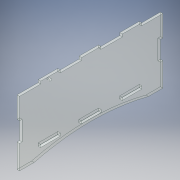
# Autodesk Inventor part: Enclosure Back
Saved by Autodesk Inventor 2018 (Build 220112000, 112)
## iProperties
Created: 2017-12-06
Part Number: Enclosure Back
Material: Glass
Document SubType Name: Modeling
Designer: Andrew
Density: 2.18 g/cm^3
Appearance: Clear
Author: Andrew
Autodesk Inventor part; units mm, degrees
ref_plane "YZ Plane" through (0, 0, 0) normal (1, 0, 0) x (0, 1, 0)
ref_plane "XZ Plane" through (0, 0, 0) normal (0, 1, 0) x (-1, 0, 0)
ref_plane "XY Plane" through (0, 0, 0) normal (0, 0, 1) x (1, 0, 0)
derived "Enclosure Top.ipt"
sketch "Sketch2" plane through (0, 0, 0) normal (0, 1, 0) x (-1, 0, 0)
  line L0 (-41.402, 93.7895) -> (-41.402, -93.7895)
  line L1 (-41.402, -93.7895) -> (41.402, -93.7895)
  line L2 (41.402, -93.7895) -> (41.402, 93.7895)
  line L3 (41.402, 93.7895) -> (-41.402, 93.7895)
  line L4 (33.576, -93.7895) -> (7.826, -93.7895)
  line L5 (7.826, -93.7895) -> (7.826, -90.4875)
  line L6 (7.826, -90.4875) -> (33.576, -90.4875)
  line L7 (33.576, -90.4875) -> (33.576, -93.7895)
  line L8 (-7.826, -93.7895) -> (-33.576, -93.7895)
  line L9 (-33.576, -93.7895) -> (-33.576, -90.4875)
  line L10 (-33.576, -90.4875) -> (-7.826, -90.4875)
  line L11 (-7.826, -90.4875) -> (-7.826, -93.7895)
  line L12 (0, -131.3053) -> (0, 131.3053)
  line L13 (-66.8528, 0) -> (66.8528, 0)
  line L14 (-41.402, -66.2073) -> (-38.1, -66.2073)
  line L15 (-38.1, -66.2073) -> (-38.1, -40.4572)
  line L16 (-38.1, -40.4572) -> (-41.402, -40.4572)
  line L17 (-41.402, -40.4572) -> (-41.402, -66.2073)
  line L18 (-41.402, -12.875) -> (-38.1, -12.875)
  line L19 (-38.1, -12.875) -> (-38.1, 12.875)
  line L20 (-38.1, 12.875) -> (-41.402, 12.875)
  line L21 (-41.402, 12.875) -> (-41.402, -12.875)
  line L22 (-41.402, 40.4572) -> (-38.1, 40.4572)
  line L23 (-38.1, 40.4572) -> (-38.1, 66.2073)
  line L24 (-38.1, 66.2073) -> (-41.402, 66.2073)
  line L25 (-41.402, 66.2073) -> (-41.402, 40.4572)
  line L26 (38.1, 50.3478) -> (36.5506, 50.3477)
  line L27 (36.5506, 50.3477) -> (36.5506, 56.3167)
  line L28 (36.5506, 56.3167) -> (38.1, 56.3167)
  line L29 (38.1, 56.3167) -> (38.1, 50.3478)
  point P0 (0, 0)
  point P1 (20.701, -90.4875)
  point P2 (-38.1, -53.3322)
  point P3 (36.5506, 53.3322)
  point P4 (-38.1, 53.3322)
sketch "Sketch3" plane through (0, 0, 0) normal (1, 0, 0) x (0, 1, 0)
  line L0 (0, 93.7895) -> (0, -93.7895) projected
  line L1 (0, 93.7895) -> (-87.817, 93.7895)
  line L2 (-87.817, -93.7895) -> (0, -93.7895)
  line L3 (-3.302, 93.7895) -> (-3.302, -93.7895) construction
  line L4 (-71.592, 93.7895) -> (-71.592, -93.7895) construction
  line L5 (-75.117, 93.7895) -> (-75.117, -93.7895) construction
  line L6 (-87.817, 93.7895) -> (-87.817, 74.7395)
  line L7 (-87.817, -93.7895) -> (-87.817, -74.7395)
  arc A0 (-87.817, -74.7395) -> (-87.817, 74.7395) centre (-376.2825, 0) ccw
  line L8 (-71.592, 66.2073) -> (-75.117, 66.2073)
  line L9 (-75.117, 66.2073) -> (-75.117, 40.4573)
  line L10 (-75.117, 40.4573) -> (-71.592, 40.4573)
  line L11 (-71.592, 40.4573) -> (-71.592, 66.2073)
  line L12 (-71.592, 12.875) -> (-75.117, 12.875)
  line L13 (-75.117, 12.875) -> (-75.117, -12.875)
  line L14 (-75.117, -12.875) -> (-71.592, -12.875)
  line L15 (-71.592, -12.875) -> (-71.592, 12.875)
  line L16 (-71.592, -40.4573) -> (-75.117, -40.4573)
  line L17 (-75.117, -40.4573) -> (-75.117, -66.2073)
  line L18 (-75.117, -66.2073) -> (-71.592, -66.2073)
  line L19 (-71.592, -66.2073) -> (-71.592, -40.4573)
  line L20 (-451.5389, 0) -> (75.2565, 0) projected
  circle A1 centre (-4.826, 53.3322) radius 1.4605
  point P0 (0, 0)
  point P1 (0, -53.3322)
  point P2 (-71.592, -53.3323)
  dimension "d10" = 3.302
  dimension "d12" = 71.592
  dimension "d13" = 3.525
  dimension "d15" = 19.05
  dimension "d16" = 12.7
  dimension "d17" = 25.75
  dimension "d20" = 3.175
  dimension "d22" = 40.4573
  dimension "d23" = 2.921
  dimension "d24" = 4.826
  constraints: 38 end point, 12 point on line, 6 parallel, 6 perpendicular, 4 collinear, 4 horizontal, 2 centre point, 2 point on circle, 2 vertical, 1 horizontal alignment, 1 midpoint, 2 other
  measures "d10" distance between parallel lines of L3 L0
  measures "d12" distance between parallel lines of L4 L0
  measures "d13" distance between parallel lines of L5 L4
  measures "d15" distance of L2.start L7.end
  measures "d16" distance between parallel lines of L7 L5
  measures "d17" distance of L10.end L8.start
  measures "d20" distance edge to line of A0 L5
  measures "d22" distance from line of L1 A1.centre
  measures "d23" diameter of A1
  measures "d24" distance from line of L0 A1.centre
extrude "Extrusion1" add sketch "Sketch3" along normal blind 3.302 contours L0 L20 L15 L12 L13 A0 L6 L1 | L0 L2 L7 A0 L20 L13 L14 L15
sketch "Sketch4" plane through (0, 0, 0) normal (1, 0, 0) x (0, 1, 0)
  line L0 (-451.5389, 0) -> (75.2565, 0) projected
  line L1 (0, 93.7895) -> (-87.817, 93.7895) projected
  line L2 (-87.817, -93.7895) -> (0, -93.7895) projected
  line L3 (0, 93.7895) -> (0, -93.7895) projected
  line L4 (0, -40.6323) -> (-3.302, -40.6323)
  line L5 (-3.302, -40.6323) -> (-3.302, -12.7)
  line L6 (-3.302, -12.7) -> (0, -12.7)
  line L7 (0, -12.7) -> (0, -40.6323)
  line L8 (0, -66.0323) -> (-3.302, -66.0323)
  line L9 (-3.302, -66.0323) -> (-3.302, -93.7895)
  line L10 (-3.302, -93.7895) -> (0, -93.7895)
  line L11 (0, -93.7895) -> (0, -66.0323)
  line L12 (0, 12.7) -> (-3.302, 12.7)
  line L13 (-3.302, 12.7) -> (-3.302, 40.6323)
  line L14 (-3.302, 40.6323) -> (0, 40.6323)
  line L15 (0, 40.6323) -> (0, 12.7)
  line L16 (0, 66.0323) -> (-3.302, 66.0323)
  line L17 (-3.302, 66.0323) -> (-3.302, 93.7895)
  line L18 (-3.302, 93.7895) -> (0, 93.7895)
  line L19 (0, 93.7895) -> (0, 66.0323)
  line L20 (-87.817, -93.7895) -> (-87.817, -74.7395) projected
  arc A0 (-87.817, -74.7395) -> (-87.817, 74.7395) centre (-376.2825, 0) ccw projected
  line L21 (-87.817, 93.7895) -> (-87.817, 74.7395) projected
  line L22 (-31.0335, 93.7895) -> (-56.7835, 93.7895)
  line L23 (-56.7835, 93.7895) -> (-56.7835, 90.4875)
  line L24 (-56.7835, 90.4875) -> (-31.0335, 90.4875)
  line L25 (-31.0335, 90.4875) -> (-31.0335, 93.7895)
  line L26 (-71.592, 93.7895) -> (-71.592, -93.7895) construction
  line L27 (-75.117, 93.7895) -> (-75.117, -93.7895) construction
  line L28 (-31.0335, -93.7895) -> (-56.7835, -93.7895)
  line L29 (-56.7835, -93.7895) -> (-56.7835, -90.4875)
  line L30 (-56.7835, -90.4875) -> (-31.0335, -90.4875)
  line L31 (-31.0335, -90.4875) -> (-31.0335, -93.7895)
  point P0 (0, 0)
  point P1 (0, -53.3322)
  point P2 (-43.9085, 90.4875)
  point P3 (-43.9085, 93.7895)
  dimension "d4" = 25.4
  dimension "d5" = 25.4
  dimension "d6" = 25.4
  dimension "d7" = 3.302
  dimension "d8" = 12.7
  dimension "d21" = 25.75
  constraints: 48 end point, 12 parallel, 10 point on line, 8 perpendicular, 6 horizontal, 3 collinear, 2 midpoint, 1 vertical alignment, 2 other
  measures "d4" distance between parallel lines of L16 L14
  measures "d5" distance between parallel lines of L6 L12
  measures "d6" distance between parallel lines of L8 L4
  measures "d7" distance of L16.start L16.end
  measures "d8" distance from line of point (0, -53.332) L4
  measures "d21" distance of L23.end L24.end
derived "Wood Rail.ipt"
extrude "Extrusion2" cut sketch "Sketch4" along normal blind 3.302 contours L12 L13 L14 L3 | L3 L4 L5 L6 | L29 L30 L31 L2 | L1 L25 L24 L23 | L16 L17 L1 L3 | L3 L2 L9 L8
equation "\"d10\" = encThick"
equation "\"d12\" = woodThickness + legHeight"
equation "\"d22\" = antOffset"
equation "\"d2\" = encThick"
equation "\"d4\" = encTab"
equation "\"d5\" = d4"
equation "\"d6\" = d5"
equation "\"d7\" = encThick"
equation "\"d8\" = 0.5 * d6"
equation "\"d18\" = encThick"
equation "\"encThick\" = 3.302"
equation "\"woodThickness\" = 3.175"
equation "\"legHeight\" = 68.416986"
equation "\"antOffset\" = 40.45725"
equation "\"encTab\" = 25.4"
body "Solid1"
